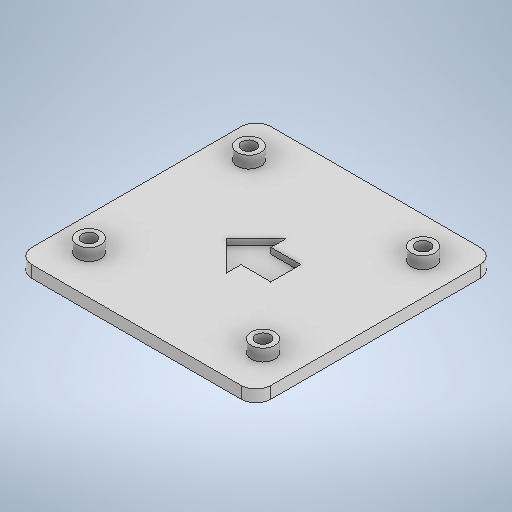
# Autodesk Inventor part: Pump Jig V1
Saved by Autodesk Inventor 2025.1 (Build 291241020, 241B)
## iProperties
Created: 2024-10-19
Part Number: Pump Jig V1
Material: Generic
Document SubType Name: Modeling
Designer: dpseu
Density: 1 g/cm^3
Appearance: Default
Author: dpseu
Autodesk Inventor part; units mm, degrees
ref_plane "YZ Plane" through (0, 0, 0) normal (1, 0, 0) x (0, 1, 0)
ref_plane "XZ Plane" through (0, 0, 0) normal (0, 1, 0) x (-1, 0, 0)
ref_plane "XY Plane" through (0, 0, 0) normal (0, 0, 1) x (1, 0, 0)
sketch "Sketch1" plane through (0, 0, 0) normal (0, 1, 0) x (-1, 0, 0)
  line L0 (0, 0) -> (-50.8, 0)
  line L1 (-50.8, 0) -> (-50.8, -50.8)
  line L2 (-50.8, -50.8) -> (0, -50.8)
  line L3 (0, -50.8) -> (0, 0)
  circle A0 centre (-6.8961, -8.4053) radius 1.5
  circle A1 centre (-6.8961, -42.4053) radius 1.5
  circle A2 centre (-6.8961, -42.4053) radius 2.5
  circle A3 centre (-6.8961, -8.4053) radius 2.5
  circle A4 centre (-43.8961, -8.3947) radius 1.4986
  circle A5 centre (-43.8961, -42.4053) radius 1.4986
  circle A6 centre (-43.8961, -42.4053) radius 2.5019
  circle A7 centre (-43.8961, -8.3947) radius 2.5019
  dimension "d9" = 50.8
  dimension "d10" = 50.8
  dimension "d11" = 3
  dimension "d12" = 3
  dimension "d13" = 34
  dimension "d14" = 5
  dimension "d15" = 5
  dimension "d16" = 8.3947
  dimension "d17" = 2.9972
  dimension "d18" = 2.9972
  dimension "d19" = 5.0038
  dimension "d20" = 5.0038
  dimension "d21" = 34.0106
  dimension "d22" = 37
  dimension "d23" = 37
  dimension "d24" = 6.8961
  constraints: 8 centre point, 8 end point, 4 coincident, 2 parallel, 1 horizontal, 1 perpendicular
  measures "d9" distance of L2.end L1.end
  measures "d10" distance of L1.end L0.end
  measures "d11" diameter of A0
  measures "d12" diameter of A1
  measures "d13" distance of A1.centre A0.centre
  measures "d14" diameter of A2
  measures "d15" diameter of A3
  measures "d16" distance from line of L2 A1.centre
  measures "d17" diameter of A4
  measures "d18" diameter of A5
  measures "d19" diameter of A6
  measures "d20" diameter of A7
  measures "d21" distance of A5.centre A4.centre
  measures "d22" distance of A4.centre A0.centre
  measures "d23" distance of A1.centre A5.centre
  measures "d24" distance from line of L3 A2.centre
extrude "Extrusion1" add sketch "Sketch1" along normal blind 2.54 contours L3 L2 L1 L0
extrude "Extrusion2" add sketch "Sketch1" along normal blind 5.08 contours A2 | A3 | A6 | A7
fillet "Fillet1" radius 3.175 4 edges at (0, 1.27, -50.8) (50.8, 1.27, -50.8) (50.8, 1.27, 0) (0, 1.27, 0)
sketch "Sketch3" plane through (0, 2.54, 0) normal (0, 1, 0) x (1, 0, 0)
  line L0 (25.4, 22.225) -> (31.75, 22.225)
  line L1 (31.75, 22.225) -> (31.75, 28.575)
  line L2 (31.75, 28.575) -> (25.4, 28.575)
  line L3 (25.4, 28.575) -> (25.4, 31.75)
  line L4 (25.4, 31.75) -> (19.05, 25.4)
  line L5 (19.05, 25.4) -> (25.4, 19.05)
  line L6 (25.4, 19.05) -> (25.4, 22.225)
  line L7 (47.625, 50.8) -> (3.175, 50.8) projected
  line L8 (0, 47.625) -> (0, 3.175) projected
  point P0 (0, 0)
  point P1 (25.4, 20.6375)
  dimension "d40" = 6.35
  dimension "d41" = 6.35
  dimension "d42" = 6.35
  dimension "d43" = 3.175
  dimension "d44" = 45
  dimension "d45" = 22.225
  dimension "d47" = 6.35
  dimension "d48" = 19.05
  constraints: 14 end point, 4 perpendicular, 1 horizontal, 1 midpoint, 1 point on line
  measures "d40" distance of L0.start L0.end
  measures "d41" distance of L0.end L1.end
  measures "d42" distance of L1.end L2.end
  measures "d43" distance of L2.end L3.end
  measures "d44" angle of L4 L3
  measures "d45" distance between parallel lines of L7 L2
  measures "d47" horizontal distance of L4.end point (25.4, 20.637)
  measures "d48" distance from line of L8 L4.end
extrude "Extrusion4" cut sketch "Sketch3" against normal blind 1.27
body "Solid1"
